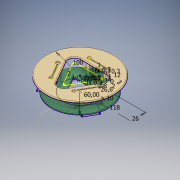
# Autodesk Inventor part: Stewart-Plate-inside
Saved by Autodesk Inventor 2018.2 (Build 222227000, 227)
## iProperties
Created: 2018-02-18
Part Number: Stewart-Plate-inside
Material: Generisch
Document SubType Name: Modeling
Designer: JochenAlt
Density: 1 g/cm^3
Appearance: Vorgabe
Author: JochenAlt
Autodesk Inventor part; units mm, degrees
ref_plane "YZ Plane" through (0, 0, 0) normal (1, 0, 0) x (0, 1, 0)
ref_plane "XZ Plane" through (0, 0, 0) normal (0, 1, 0) x (-1, 0, 0)
sketch "Skizze1" plane through (0, 0, 0) normal (0, 0, 1) x (1, 0, 0)
  line L0 (-9.8, 0) -> (9.8, 0) construction
  line L1 (-7, 36) -> (7, 36)
  line L2 (7, 36) -> (7, 33)
  line L3 (7, 33) -> (-7, 33)
  line L4 (-7, 33) -> (-7, 36)
  line L5 (1.5, 33) -> (-1.5, 33)
  line L6 (-1.5, 33) -> (-1.5, 28)
  line L7 (-1.5, 28) -> (1.5, 28)
  line L8 (1.5, 28) -> (1.5, 33)
  line L9 (0, 43.2) -> (0, -7.2) construction
  point P0 (0, 0)
  dimension "d10" = 3
  dimension "d14" = 14
  dimension "d23" = 5
  constraints: 16 end point, 4 parallel, 3 perpendicular, 2 horizontal, 2 point on line, 1 midpoint, 1 other
  measures "d10" distance between parallel lines of L3 L1
  measures "d14" distance between parallel lines of L2 L4
  measures "d23" distance between parallel lines of L3 L7
extrude "Extrusion3" add sketch "Skizze1" against normal blind 7
fillet "Rundung1" radius 4 2 edges at (-7, 34.5, -7) (7, 34.5, -7)
sketch "Skizze2" plane through (-7, 36, 0) normal (0, 1, 0) x (1, 0, 0)
  circle A0 centre (3, 4) radius 1.1
  circle A1 centre (11, 4) radius 1.1
  line L0 (7, 0) -> (7, 7) construction
  line L1 (43, 0) -> (-27, 0) construction
  line L2 (-1.6221, 4) -> (19.0112, 4) construction
  line L3 (0, 7) -> (14, 7) construction
  line L4 (0, 0) -> (0, 7) projected
  point P0 (4, 7)
  point P1 (10, 7)
  point P2 (0, 3)
  dimension "d16" = 2.2
  dimension "d20" = 3
  dimension "d21" = 3
  constraints: 4 end point, 2 centre point, 1 equal radius, 1 horizontal, 1 midpoint, 1 point on line, 1 symmetric about line, 1 vertical
  measures "d16" diameter of A0
  measures "d20" distance between parallel lines of L3 L2
  measures "d21" distance from line of L4 A0.centre
extrude "Extrusion4" cut sketch "Skizze2" against normal up to next
chamfer "Fase1" distance 5 distance2 7 1 edges at (0, 28, -7) measured on face at (0, 28.5, -7)
pattern_circular "Runde Anordnung1" count 3 over 360 about axis through (0, 0, -10) along (0, 0, 1) of "Extrusion3", "Extrusion4", "Fase1", "Rundung1"
sketch "Skizze3" plane through (0, 0, 0) normal (0, 0, 1) x (1, 0, 0)
  line L0 (0, 73.7285) -> (0, -70.6214) construction
  circle A0 centre (0, 0) radius 50
  line L1 (23.7291, 15.7) -> (-23.7291, 15.7)
  line L2 (-25.4611, 12.7) -> (-1.7321, -28.4)
  line L3 (25.4611, 12.7) -> (1.7321, -28.4)
  line L4 (-11.5394, 6.6623) -> (13.5966, -7.85) construction
  line L5 (27.1932, 15.7) -> (-13.5966, -7.85) construction
  line L6 (0.15, 52.6) -> (12.15, 52.6) construction
  line L7 (12.15, 52.6) -> (12.15, 26) construction
  line L8 (12.15, 26) -> (0.15, 26) construction
  line L9 (0.15, 26) -> (0.15, 52.6) construction
  line L10 (-0.15, 52.6) -> (-12.15, 52.6) construction
  line L11 (-12.15, 52.6) -> (-12.15, 26) construction
  line L12 (-12.15, 26) -> (-0.15, 26) construction
  line L13 (-0.15, 26) -> (-0.15, 52.6) construction
  line L14 (11.45, 25.7) -> (-11.45, 25.7)
  arc A1 (-23.7291, 15.7) -> (-25.4611, 12.7) centre (-23.7291, 13.7) ccw
  arc A2 (-1.7321, -28.4) -> (1.7321, -28.4) centre (0, -27.4) ccw
  arc A3 (25.4611, 12.7) -> (23.7291, 15.7) centre (23.7291, 13.7) ccw
  line L15 (-12.45, 31.5) -> (12.45, 31.5) construction
  line L16 (12.45, 32.7) -> (-12.45, 32.7) construction
  line L17 (-12.45, 31.2) -> (12.45, 31.2)
  line L18 (-12.45, 33) -> (12.45, 33)
  line L19 (-12.45, 26.7) -> (-12.45, 51.9)
  line L20 (-11.45, 52.9) -> (11.45, 52.9)
  line L21 (12.45, 51.9) -> (12.45, 26.7)
  arc A4 (-11.45, 52.9) -> (-12.45, 51.9) centre (-11.45, 51.9) ccw
  arc A5 (12.45, 51.9) -> (11.45, 52.9) centre (11.45, 51.9) ccw
  arc A6 (11.45, 25.7) -> (12.45, 26.7) centre (11.45, 26.7) ccw
  arc A7 (-12.45, 26.7) -> (-11.45, 25.7) centre (-11.45, 26.7) ccw
  line L22 (-12.45, 35.15) -> (12.45, 35.15) construction
  circle A8 centre (0, 0) radius 36.7791 construction
  circle A9 centre (-16.6, 32.8198) radius 2.15 construction
  line L23 (-14.3846, 33.9403) -> (-14.5219, 31.4615)
  line L24 (-14.5219, 31.4615) -> (-16.7373, 30.341)
  line L25 (-16.7373, 30.341) -> (-18.8154, 31.6993)
  line L26 (-18.8154, 31.6993) -> (-18.6781, 34.1781)
  line L27 (-18.6781, 34.1781) -> (-16.4627, 35.2986)
  line L28 (-16.4627, 35.2986) -> (-14.3846, 33.9403)
  line L29 (-16.6, 32.8198) -> (-17.5704, 34.7383) construction
  line L30 (-16.6, 32.8198) -> (0, 0) construction
  line L31 (0, 0) -> (16.6, 32.8198) construction
  circle A10 centre (16.6, 32.8198) radius 2.15 construction
  line L32 (18.8154, 31.6993) -> (16.7373, 30.341)
  line L33 (16.7373, 30.341) -> (14.5219, 31.4615)
  line L34 (14.5219, 31.4615) -> (14.3846, 33.9403)
  line L35 (14.3846, 33.9403) -> (16.4627, 35.2986)
  line L36 (16.4627, 35.2986) -> (18.6781, 34.1781)
  line L37 (18.6781, 34.1781) -> (18.8154, 31.6993)
  line L38 (16.6, 32.8198) -> (17.5704, 34.7383) construction
  arc A11 (16.6, 28.6698) -> (16.6, 36.9698) centre (16.6, 32.8198) ccw
  line L39 (-12.45, 36.9698) -> (-12.45, 28.6698)
  line L40 (-12.45, 28.6698) -> (-16.6, 28.6698)
  arc A12 (-16.6, 36.9698) -> (-16.6, 28.6698) centre (-16.6, 32.8198) ccw
  line L41 (12.45, 36.9698) -> (12.45, 28.6698)
  line L42 (16.6, 36.9698) -> (12.45, 36.9698)
  line L43 (16.6, 28.6698) -> (12.45, 28.6698)
  line L44 (-12.45, 36.9698) -> (-16.6, 36.9698)
  circle A13 centre (16.6, 32.8198) radius 4.15 construction
  circle A14 centre (-16.6, 32.8198) radius 4.15 construction
  circle A15 centre (16.6, 32.8198) radius 1.4
  circle A16 centre (-16.6, 32.8198) radius 1.4
  line L45 (-16.8979, -24.132) -> (-38.7217, -36.732)
  line L46 (-40.0877, -36.366) -> (-51.5377, -16.534)
  arc A17 (-40.0877, -36.366) -> (-38.7217, -36.732) centre (-39.2217, -35.866) ccw
  arc A18 (-16.8979, -24.132) -> (-16.5319, -22.766) centre (-17.3979, -23.266) ccw
  line L47 (-27.9819, -2.934) -> (-16.5319, -22.766)
  line L48 (-20.795, -26.382) -> (-33.245, -4.818)
  line L49 (-22.3538, -27.282) -> (-34.8038, -5.718)
  line L50 (-51.1717, -15.168) -> (-29.3479, -2.568)
  line L51 (-40.3168, -4.1089) -> (-38.2418, -7.7029)
  line L52 (-36.5855, -4.5127) -> (-38.8008, -3.3922)
  line L53 (-34.5074, -3.1544) -> (-36.5855, -4.5127)
  circle A19 centre (-36.7228, -2.0339) radius 2.15 construction
  line L54 (-33.1288, 0.0411) -> (-31.0538, -3.5529)
  arc A20 (-33.1288, 0.0411) -> (-40.3168, -4.1089) centre (-36.7228, -2.0339) ccw
  line L55 (-36.8601, 0.4449) -> (-34.6447, -0.6756)
  circle A21 centre (-36.7228, -2.0339) radius 1.4
  line L56 (0, 0) -> (-36.7228, -2.0339) construction
  line L57 (-34.6447, -0.6756) -> (-34.5074, -3.1544)
  line L58 (-38.8008, -3.3922) -> (-38.9381, -0.9134)
  line L59 (-38.9381, -0.9134) -> (-36.8601, 0.4449)
  line L60 (-22.2008, -29.4276) -> (-19.9855, -28.3071)
  line L61 (-18.6038, -25.1169) -> (-16.5288, -28.7109)
  line L62 (-25.7918, -29.2669) -> (-18.6038, -25.1169)
  line L63 (-22.3381, -31.9064) -> (-22.2008, -29.4276)
  circle A22 centre (-20.1228, -30.7859) radius 1.4
  line L64 (-25.7918, -29.2669) -> (-23.7168, -32.8609)
  circle A23 centre (-20.1228, -30.7859) radius 4.15 construction
  line L65 (-17.9074, -29.6654) -> (-18.0447, -32.1442)
  line L66 (-19.9855, -28.3071) -> (-17.9074, -29.6654)
  line L67 (-18.0447, -32.1442) -> (-20.2601, -33.2647)
  arc A24 (-23.7168, -32.8609) -> (-16.5288, -28.7109) centre (-20.1228, -30.7859) ccw
  line L68 (-20.2601, -33.2647) -> (-22.3381, -31.9064)
  line L69 (-38.2418, -7.7029) -> (-31.0538, -3.5529)
  arc A25 (-27.9819, -2.934) -> (-29.3479, -2.568) centre (-28.8479, -3.434) ccw
  arc A26 (-51.1717, -15.168) -> (-51.5377, -16.534) centre (-50.6717, -16.034) ccw
  line L70 (29.3479, -2.568) -> (51.1717, -15.168)
  line L71 (51.5377, -16.534) -> (40.0877, -36.366)
  arc A27 (51.5377, -16.534) -> (51.1717, -15.168) centre (50.6717, -16.034) ccw
  arc A28 (29.3479, -2.568) -> (27.9819, -2.934) centre (28.8479, -3.434) ccw
  line L72 (16.5319, -22.766) -> (27.9819, -2.934)
  line L73 (33.245, -4.818) -> (20.795, -26.382)
  line L74 (34.8038, -5.718) -> (22.3538, -27.282)
  line L75 (38.7217, -36.732) -> (16.8979, -24.132)
  line L76 (23.7168, -32.8609) -> (25.7918, -29.2669)
  line L77 (22.2008, -29.4276) -> (22.3381, -31.9064)
  line L78 (19.9855, -28.3071) -> (22.2008, -29.4276)
  circle A29 centre (20.1228, -30.7859) radius 2.15 construction
  line L79 (16.5288, -28.7109) -> (18.6038, -25.1169)
  arc A30 (16.5288, -28.7109) -> (23.7168, -32.8609) centre (20.1228, -30.7859) ccw
  line L80 (18.0447, -32.1442) -> (17.9074, -29.6654)
  circle A31 centre (20.1228, -30.7859) radius 1.4
  line L81 (0, 0) -> (20.1228, -30.7859) construction
  line L82 (17.9074, -29.6654) -> (19.9855, -28.3071)
  line L83 (22.3381, -31.9064) -> (20.2601, -33.2647)
  line L84 (20.2601, -33.2647) -> (18.0447, -32.1442)
  line L85 (36.5855, -4.5127) -> (34.5074, -3.1544)
  line L86 (31.0538, -3.5529) -> (33.1288, 0.0411)
  line L87 (38.2418, -7.7029) -> (31.0538, -3.5529)
  line L88 (38.8008, -3.3922) -> (36.5855, -4.5127)
  circle A32 centre (36.7228, -2.0339) radius 1.4
  line L89 (38.2418, -7.7029) -> (40.3168, -4.1089)
  circle A33 centre (36.7228, -2.0339) radius 4.15 construction
  line L90 (34.6447, -0.6756) -> (36.8601, 0.4449)
  line L91 (34.5074, -3.1544) -> (34.6447, -0.6756)
  line L92 (36.8601, 0.4449) -> (38.9381, -0.9134)
  arc A34 (40.3168, -4.1089) -> (33.1288, 0.0411) centre (36.7228, -2.0339) ccw
  line L93 (38.9381, -0.9134) -> (38.8008, -3.3922)
  line L94 (25.7918, -29.2669) -> (18.6038, -25.1169)
  arc A35 (16.5319, -22.766) -> (16.8979, -24.132) centre (17.3979, -23.266) ccw
  arc A36 (38.7217, -36.732) -> (40.0877, -36.366) centre (39.2217, -35.866) ccw
  point P0 (-27.1932, 15.7)
  point P1 (0, -31.4)
  point P2 (19.75, 15.7)
  point P3 (-14.2556, 15.7)
  point P4 (-15.9349, -3.8)
  point P5 (11.2583, -11.9)
  point P6 (-4.5899, -23.45)
  point P7 (-15.4237, 34.6195)
  point P8 (18.7467, 32.9387)
  point P9 (-24.2158, -28.357)
  point P10 (-22.094, -27.132)
  point P11 (-21.0548, -26.532)
  point P12 (-36.6658, -6.793)
  point P13 (-34.544, -5.568)
  point P14 (-33.5048, -4.968)
  point P15 (-37.8991, -0.2342)
  point P16 (-38.8695, -2.1528)
  point P17 (-22.2695, -30.667)
  point P18 (-21.2991, -32.5856)
  point P19 (36.6658, -6.793)
  point P20 (34.544, -5.568)
  point P21 (33.5048, -4.968)
  point P22 (24.2158, -28.357)
  point P23 (22.094, -27.132)
  point P24 (21.0548, -26.532)
  point P25 (19.1524, -32.7045)
  point P26 (21.2991, -32.5856)
  point P27 (37.6932, -3.9524)
  point P28 (38.8695, -2.1528)
  dimension "d140" = 60
  dimension "d146" = 0.3
  dimension "d147" = 26.6
  dimension "d148" = 12
  dimension "d150" = 0.3
  dimension "d160" = 10
  dimension "d164" = 26
  dimension "d184" = 2
  dimension "d189" = 100
  dimension "d199" = 5.5
  dimension "d200" = 1.2
  dimension "d201" = 0.3
  dimension "d202" = 0.3
  dimension "d203" = 0.3
  dimension "d204" = 0.3
  dimension "d205" = 1
  dimension "d211" = 4.3
  dimension "d213" = 0
  dimension "d214" = 2
  dimension "d227" = 2.8
  dimension "d230" = 360
  constraints: 188 end point, 54 point on circle, 48 point on line, 37 centre point, 21 tangent, 11 coincident, 10 midpoint, 8 equal radius, 6 parallel, 5 horizontal, 4 collinear, 4 perpendicular, 2 symmetric about line, 2 vertical, 298 other
  measures "d140" angle of L3 L1
  measures "d146" distance between parallel lines of L9 L13
  measures "d147" distance between parallel lines of L8 L6
  measures "d148" distance between parallel lines of L7 L9
  measures "d150" distance between parallel lines of L14 L8
  measures "d160" distance between parallel lines of L1 L14
  measures "d164" distance from line of point (0, 0) L8
  measures "d184" radius of A1
  measures "d189" diameter of A0
  measures "d199" distance between parallel lines of L15 L12
  measures "d200" distance between parallel lines of L16 L15
  measures "d201" distance between parallel lines of L17 L15
  measures "d202" distance between parallel lines of L16 L18
  measures "d203" distance between parallel lines of L6 L20
  measures "d204" distance between parallel lines of L11 L19
  measures "d205" radius of A4
  measures "d211" diameter of A9
  measures "d213" distance between parallel lines of L21 L41
  measures "d214" radial gap between concentric circles of A13 A10
  measures "d227" diameter of A15
extrude "Extrusion11" add sketch "Skizze3" along normal blind 2.5 contours A0 L70 L89 A34 L86 A28 L72 A35 L75 L79 A30 L76 L45 L64 A24 L61 A18 L47 A25 L50 L54 A20 L51 L19 L44 A12 L40 A7 L14 A6 L21 L43 A11 L42 | L21 L18 L19 A0 | A0 L75 L74 L70 | L42 A11 L43 L21 | L70 L86 A34 L89 | L50 L49 L45 A0 | L19 L40 A12 L44 | L76 A30 L79 L75 | L51 A20 L54 L50 | L21 A6 L14 A7 L19 L17 | L45 L61 A24 L64 | L73 L75 A35 L72 A28 L70 | L50 A25 L47 A18 L45 L48 | L23 L24 L25 L26 L27 L28 | L32 L33 L34 L35 L36 L37 | L52 L58 L59 L55 L57 L53 | L60 L66 L65 L67 L68 L63 | L77 L83 L84 L80 L82 L78 | L85 L91 L90 L92 L93 L88
extrude "Extrusion9" cut sketch "Skizze3" against normal blind 1 from surface at 2.5 contours L21 L18 L19 A0 | A0 L19 A4 L20 A5 L21 | L70 A27 L71 A36 L75 A0 | A0 L75 L74 L70 | L50 L49 L45 A0 | A0 L45 A17 L46 A26 L50 | L21 A6 L14 A7 L19 L17 | L73 L75 A35 L72 A28 L70 | L50 A25 L47 A18 L45 L48 | A3 L3 A2 L2 A1 L1
fillet "Rundung4" radius 1 17 edges at (0, -50, 2.5) (49.5385, -6.7778, 2.5) (39.5127, 30.639, 2.5) (-43.3013, 25, 2.5) (-50, 0, 0) (25.4611, 14.7, 2.5) (13.5966, -7.85, 2.5) (0, -29.4, 2.5) (-13.5966, -7.85, 2.5) (-25.4611, 14.7, 2.5) (0, 15.7, 2.5) (-25.4611, 14.7, 0) (-13.5966, -7.85, 0) (0, -29.4, 0) (13.5966, -7.85, 0) (25.4611, 14.7, 0) (0, 15.7, 0)
fillet "Rundung4" radius 0.75 7 edges at (-12.45, 40.7126, 1.5) (-12.1571, 25.9929, 1.5) (0, 25.7, 1.5) (12.1571, 25.9929, 1.5) (12.45, 28.95, 1.5) (-12.45, 28.95, 1.5) (12.45, 40.7126, 1.5)
extrude "Extrusion14" add sketch "Skizze3" along normal blind 13 contours L42 A11 L43 L21 | L70 L86 A34 L89 | L19 L40 A12 L44 | L76 A30 L79 L75 | L51 A20 L54 L50 | L45 L61 A24 L64 | L23 L24 L25 L26 L27 L28 | L32 L33 L34 L35 L36 L37 | L52 L58 L59 L55 L57 L53 | L60 L66 L65 L67 L68 L63 | L77 L83 L84 L80 L82 L78 | L85 L91 L90 L92 L93 L88
extrude "Extrusion15" cut sketch "Skizze3" against normal blind 6 from surface at 13 contours L23 L24 L25 L26 L27 L28 | L32 L33 L34 L35 L36 L37 | A15 | A16 | L52 L58 L59 L55 L57 L53 | L60 L66 L65 L67 L68 L63 | L77 L83 L84 L80 L82 L78 | L85 L91 L90 L92 L93 L88
ref_plane "Arbeitsebene1" through (0, 0, 24.5) normal (0, 0, 1) x (1, 0, 0)
sketch "Skizze8" plane through (0, 0, 24.5) normal (0, 0, 1) x (1, 0, 0)
  circle A0 centre (36.7228, -2.0339) radius 1.4 projected
  circle A1 centre (20.1228, -30.7859) radius 1.4 projected
  circle A2 centre (-20.1228, -30.7859) radius 1.4 projected
  circle A3 centre (-36.7228, -2.0339) radius 1.4 projected
  circle A4 centre (-16.6, 32.8198) radius 1.4 projected
  circle A5 centre (16.6, 32.8198) radius 1.4 projected
  line L0 (18.6781, 34.1781) -> (18.8154, 31.6993) projected
  line L1 (16.4627, 35.2986) -> (18.6781, 34.1781) projected
  line L2 (14.3846, 33.9403) -> (16.4627, 35.2986) projected
  line L3 (14.5219, 31.4615) -> (14.3846, 33.9403) projected
  line L4 (16.7373, 30.341) -> (14.5219, 31.4615) projected
  line L5 (18.8154, 31.6993) -> (16.7373, 30.341) projected
  circle A6 centre (-16.6, 32.8198) radius 1.4 projected
  line L6 (-16.4627, 35.2986) -> (-14.3846, 33.9403) projected
  line L7 (-18.6781, 34.1781) -> (-16.4627, 35.2986) projected
  line L8 (-18.8154, 31.6993) -> (-18.6781, 34.1781) projected
  line L9 (-16.7373, 30.341) -> (-18.8154, 31.6993) projected
  line L10 (-14.5219, 31.4615) -> (-16.7373, 30.341) projected
  line L11 (-14.3846, 33.9403) -> (-14.5219, 31.4615) projected
  circle A7 centre (-36.7228, -2.0339) radius 1.4 projected
  line L12 (-34.6447, -0.6756) -> (-34.5074, -3.1544) projected
  line L13 (-36.8601, 0.4449) -> (-34.6447, -0.6756) projected
  line L14 (-38.9381, -0.9134) -> (-36.8601, 0.4449) projected
  line L15 (-38.8008, -3.3922) -> (-38.9381, -0.9134) projected
  line L16 (-36.5855, -4.5127) -> (-38.8008, -3.3922) projected
  line L17 (-34.5074, -3.1544) -> (-36.5855, -4.5127) projected
  circle A8 centre (36.7228, -2.0339) radius 1.4 projected
  line L18 (38.8008, -3.3922) -> (36.5855, -4.5127) projected
  line L19 (38.9381, -0.9134) -> (38.8008, -3.3922) projected
  line L20 (36.8601, 0.4449) -> (38.9381, -0.9134) projected
  line L21 (34.6447, -0.6756) -> (36.8601, 0.4449) projected
  line L22 (34.5074, -3.1544) -> (34.6447, -0.6756) projected
  line L23 (36.5855, -4.5127) -> (34.5074, -3.1544) projected
  circle A9 centre (20.1228, -30.7859) radius 1.4 projected
  line L24 (17.9074, -29.6654) -> (19.9855, -28.3071) projected
  line L25 (18.0447, -32.1442) -> (17.9074, -29.6654) projected
  line L26 (20.2601, -33.2647) -> (18.0447, -32.1442) projected
  line L27 (22.3381, -31.9064) -> (20.2601, -33.2647) projected
  line L28 (22.2008, -29.4276) -> (22.3381, -31.9064) projected
  line L29 (19.9855, -28.3071) -> (22.2008, -29.4276) projected
  circle A10 centre (-20.1228, -30.7859) radius 1.4 projected
  line L30 (-22.3381, -31.9064) -> (-22.2008, -29.4276) projected
  line L31 (-20.2601, -33.2647) -> (-22.3381, -31.9064) projected
  line L32 (-18.0447, -32.1442) -> (-20.2601, -33.2647) projected
  line L33 (-17.9074, -29.6654) -> (-18.0447, -32.1442) projected
  line L34 (-19.9855, -28.3071) -> (-17.9074, -29.6654) projected
  line L35 (-22.2008, -29.4276) -> (-19.9855, -28.3071) projected
  line L36 (-22.3381, -31.9064) -> (-22.2008, -29.4276) projected
  line L37 (-22.2008, -29.4276) -> (-19.9855, -28.3071) projected
  line L38 (-19.9855, -28.3071) -> (-17.9074, -29.6654) projected
  line L39 (-17.9074, -29.6654) -> (-18.0447, -32.1442) projected
  line L40 (-18.0447, -32.1442) -> (-20.2601, -33.2647) projected
  line L41 (-20.2601, -33.2647) -> (-22.3381, -31.9064) projected
  line L42 (-18.6038, -25.1169) -> (-25.7918, -29.2669) projected
  line L43 (-25.7918, -29.2669) -> (-23.7168, -32.8609) projected
  arc A11 (-23.7168, -32.8609) -> (-16.5288, -28.7109) centre (-20.1228, -30.7859) ccw projected
  line L44 (-16.5288, -28.7109) -> (-18.6038, -25.1169) projected
  line L45 (-34.6447, -0.6756) -> (-34.5074, -3.1544) projected
  line L46 (-34.5074, -3.1544) -> (-36.5855, -4.5127) projected
  line L47 (-36.5855, -4.5127) -> (-38.8008, -3.3922) projected
  line L48 (-38.8008, -3.3922) -> (-38.9381, -0.9134) projected
  line L49 (-38.9381, -0.9134) -> (-36.8601, 0.4449) projected
  line L50 (-36.8601, 0.4449) -> (-34.6447, -0.6756) projected
  line L51 (-40.3168, -4.1089) -> (-38.2418, -7.7029) projected
  line L52 (-38.2418, -7.7029) -> (-31.0538, -3.5529) projected
  line L53 (-31.0538, -3.5529) -> (-33.1288, 0.0411) projected
  arc A12 (-33.1288, 0.0411) -> (-40.3168, -4.1089) centre (-36.7228, -2.0339) ccw projected
  line L54 (17.9074, -29.6654) -> (19.9855, -28.3071) projected
  line L55 (19.9855, -28.3071) -> (22.2008, -29.4276) projected
  line L56 (22.2008, -29.4276) -> (22.3381, -31.9064) projected
  line L57 (22.3381, -31.9064) -> (20.2601, -33.2647) projected
  line L58 (20.2601, -33.2647) -> (18.0447, -32.1442) projected
  line L59 (18.0447, -32.1442) -> (17.9074, -29.6654) projected
  line L60 (23.7168, -32.8609) -> (25.7918, -29.2669) projected
  line L61 (25.7918, -29.2669) -> (18.6038, -25.1169) projected
  line L62 (18.6038, -25.1169) -> (16.5288, -28.7109) projected
  arc A13 (16.5288, -28.7109) -> (23.7168, -32.8609) centre (20.1228, -30.7859) ccw projected
  line L63 (38.8008, -3.3922) -> (36.5855, -4.5127) projected
  line L64 (36.5855, -4.5127) -> (34.5074, -3.1544) projected
  line L65 (34.5074, -3.1544) -> (34.6447, -0.6756) projected
  line L66 (34.6447, -0.6756) -> (36.8601, 0.4449) projected
  line L67 (36.8601, 0.4449) -> (38.9381, -0.9134) projected
  line L68 (38.9381, -0.9134) -> (38.8008, -3.3922) projected
  line L69 (31.0538, -3.5529) -> (38.2418, -7.7029) projected
  line L70 (38.2418, -7.7029) -> (40.3168, -4.1089) projected
  arc A14 (40.3168, -4.1089) -> (33.1288, 0.0411) centre (36.7228, -2.0339) ccw projected
  line L71 (33.1288, 0.0411) -> (31.0538, -3.5529) projected
  line L72 (18.6781, 34.1781) -> (18.8154, 31.6993) projected
  line L73 (18.8154, 31.6993) -> (16.7373, 30.341) projected
  line L74 (16.7373, 30.341) -> (14.5219, 31.4615) projected
  line L75 (14.5219, 31.4615) -> (14.3846, 33.9403) projected
  line L76 (14.3846, 33.9403) -> (16.4627, 35.2986) projected
  line L77 (16.4627, 35.2986) -> (18.6781, 34.1781) projected
  line L78 (12.45, 36.9698) -> (12.45, 28.6698) projected
  line L79 (12.45, 28.6698) -> (16.6, 28.6698) projected
  arc A15 (16.6, 28.6698) -> (16.6, 36.9698) centre (16.6, 32.8198) ccw projected
  line L80 (16.6, 36.9698) -> (12.45, 36.9698) projected
  line L81 (-16.4627, 35.2986) -> (-14.3846, 33.9403) projected
  line L82 (-14.3846, 33.9403) -> (-14.5219, 31.4615) projected
  line L83 (-14.5219, 31.4615) -> (-16.7373, 30.341) projected
  line L84 (-16.7373, 30.341) -> (-18.8154, 31.6993) projected
  line L85 (-18.8154, 31.6993) -> (-18.6781, 34.1781) projected
  line L86 (-18.6781, 34.1781) -> (-16.4627, 35.2986) projected
  line L87 (-12.45, 28.6698) -> (-12.45, 36.9698) projected
  line L88 (-12.45, 36.9698) -> (-16.6, 36.9698) projected
  arc A16 (-16.6, 36.9698) -> (-16.6, 28.6698) centre (-16.6, 32.8198) ccw projected
  line L89 (-16.6, 28.6698) -> (-12.45, 28.6698) projected
  circle A17 centre (0, 0) radius 59
  line L90 (51.5377, -16.534) -> (40.0877, -36.366) projected
  arc A18 (38.7217, -36.732) -> (40.0877, -36.366) centre (39.2217, -35.866) ccw projected
  line L91 (38.7217, -36.732) -> (16.8979, -24.132) projected
  line L92 (34.8038, -5.718) -> (22.3538, -27.282) projected
  line L93 (33.245, -4.818) -> (20.795, -26.382) projected
  line L94 (16.5319, -22.766) -> (27.9819, -2.934) projected
  arc A19 (16.5319, -22.766) -> (16.8979, -24.132) centre (17.3979, -23.266) ccw projected
  line L95 (29.3479, -2.568) -> (51.1717, -15.168) projected
  arc A20 (29.3479, -2.568) -> (27.9819, -2.934) centre (28.8479, -3.434) ccw projected
  arc A21 (51.5377, -16.534) -> (51.1717, -15.168) centre (50.6717, -16.034) ccw projected
  line L96 (-27.9819, -2.934) -> (-16.5319, -22.766) projected
  arc A22 (-16.8979, -24.132) -> (-16.5319, -22.766) centre (-17.3979, -23.266) ccw projected
  line L97 (-16.8979, -24.132) -> (-38.7217, -36.732) projected
  arc A23 (-40.0877, -36.366) -> (-38.7217, -36.732) centre (-39.2217, -35.866) ccw projected
  line L98 (-40.0877, -36.366) -> (-51.5377, -16.534) projected
  arc A24 (-51.1717, -15.168) -> (-51.5377, -16.534) centre (-50.6717, -16.034) ccw projected
  line L99 (-51.1717, -15.168) -> (-29.3479, -2.568) projected
  arc A25 (-27.9819, -2.934) -> (-29.3479, -2.568) centre (-28.8479, -3.434) ccw projected
  line L100 (-12.45, 26.7) -> (-12.45, 51.9) projected
  line L101 (-11.45, 52.9) -> (11.45, 52.9) projected
  line L102 (12.45, 51.9) -> (12.45, 26.7) projected
  arc A26 (12.45, 51.9) -> (11.45, 52.9) centre (11.45, 51.9) ccw projected
  arc A27 (-11.45, 52.9) -> (-12.45, 51.9) centre (-11.45, 51.9) ccw projected
  arc A28 (11.45, 25.7) -> (12.45, 26.7) centre (11.45, 26.7) ccw projected
  line L103 (11.45, 25.7) -> (-11.45, 25.7) projected
  arc A29 (-12.45, 26.7) -> (-11.45, 25.7) centre (-11.45, 26.7) ccw projected
  line L104 (-12.45, 33) -> (12.45, 33) projected
  line L105 (-12.45, 31.2) -> (12.45, 31.2) projected
  line L106 (-20.795, -26.382) -> (-33.245, -4.818) projected
  line L107 (-22.3538, -27.282) -> (-34.8038, -5.718) projected
  line L108 (25.4611, 12.7) -> (1.7321, -28.4) projected
  arc A30 (-1.7321, -28.4) -> (1.7321, -28.4) centre (0, -27.4) ccw projected
  line L109 (-25.4611, 12.7) -> (-1.7321, -28.4) projected
  arc A31 (25.4611, 12.7) -> (23.7291, 15.7) centre (23.7291, 13.7) ccw projected
  line L110 (23.7291, 15.7) -> (-23.7291, 15.7) projected
  arc A32 (-23.7291, 15.7) -> (-25.4611, 12.7) centre (-23.7291, 13.7) ccw projected
  line L111 (-23.7291, 24.7) -> (23.7291, 24.7)
  arc A33 (33.2554, 8.2) -> (23.7291, 24.7) centre (23.7291, 13.7) ccw
  line L112 (33.2554, 8.2) -> (9.5263, -32.9)
  arc A34 (-9.5263, -32.9) -> (9.5263, -32.9) centre (0, -27.4) ccw
  line L113 (-9.5263, -32.9) -> (-33.2554, 8.2)
  arc A35 (-23.7291, 24.7) -> (-33.2554, 8.2) centre (-23.7291, 13.7) ccw
  dimension "d236" = 118
  dimension "d251" = 1
  constraints: 6 end point, 6 point on circle, 4 centre point, 1 coincident, 5 other
  measures "d236" diameter of A17
  measures "d251" distance between parallel lines of L103 L111
extrude "Extrusion17" add sketch "Skizze8" along normal blind 2 separate body contours L0 L5 L4 L3 L2 L1 | L6 L11 L10 L9 L8 L7 | L12 L17 L16 L15 L14 L13 | L18 L23 L22 L21 L20 L19 | L24 L29 L28 L27 L26 L25 | L30 L35 L34 L33 L32 L31 | L44 A11 L43 L42 | L42 L106 L52 L99 A25 L96 A22 L97 | L42 L97 A23 L98 A24 L99 L52 L107 | L52 L51 A12 L53 | A13 L62 L61 L60 | L61 L92 L69 L95 A21 L90 A18 L91 | L91 A19 L94 A20 L95 L69 L93 L61 | L69 L71 A14 L70 | L80 A15 L79 L78 | L78 L104 L87 L100 A27 L101 A26 L102 | L78 L102 A28 L103 A29 L100 L87 L105 | L87 L89 A16 L88 | A17
extrude "Extrusion20" cut sketch "Skizze8" along normal blind 1 contours A0 | L42 L106 L52 L99 A25 L96 A22 L97 | L42 L107 L52 L106 | L42 L97 A23 L98 A24 L99 L52 L107 | L61 L92 L69 L95 A21 L90 A18 L91 | L61 L93 L69 L92 | L91 A19 L94 A20 L95 L69 L93 L61 | L78 L104 L87 L100 A27 L101 A26 L102 | L78 L105 L87 L104 | L78 L102 A28 L103 A29 L100 L87 L105 bodies 1 2
extrude "Extrusion18" add sketch "Skizze8" against normal up to surface (11.5 mm away) contours L6 L11 L10 L9 L8 L7 | L12 L17 L16 L15 L14 L13 | L24 L29 L28 L27 L26 L25 | L30 L35 L34 L33 L32 L31 | L44 A11 L43 L42 | L52 L51 A12 L53 | A13 L62 L61 L60 | L69 L71 A14 L70 | L80 A15 L79 L78 | L87 L89 A16 L88 bodies 2
extrude "Extrusion19" cut sketch "Skizze8" along normal blind 6 from surface at -11.5 contours L0 L5 L4 L3 L2 L1 | L6 L11 L10 L9 L8 L7 | L12 L17 L16 L15 L14 L13 | L18 L23 L22 L21 L20 L19 | L24 L29 L28 L27 L26 L25 | L30 L35 L34 L33 L32 L31 bodies 1
fillet "Rundung6" radius 1 14 edges at (-59, 0, 24.5) (-59, 0, 26.5) (33.2554, 19.2, 26.5) (21.3908, -12.35, 26.5) (0, -38.4, 26.5) (-21.3908, -12.35, 26.5) (-33.2554, 19.2, 26.5) (0, 24.7, 26.5) (-33.2554, 19.2, 24.5) (-21.3908, -12.35, 24.5) (0, -38.4, 24.5) (21.3908, -12.35, 24.5) (33.2554, 19.2, 24.5) (0, 24.7, 24.5)
fillet "Rundung6" radius 0.75 30 edges at (51.6376, -15.7752, 25.5) (45.8127, -26.45, 25.5) (39.4805, -36.8319, 25.5) (30.5378, -32.007, 25.5) (42.9878, -10.443, 25.5) (28.5891, -2.4681, 25.5) (22.2569, -12.85, 25.5) (16.432, -23.5248, 25.5) (18.8464, -25.257, 25.5) (31.2964, -3.693, 25.5) (-51.6376, -15.7752, 25.5) (-45.8127, -26.45, 25.5) (-39.4805, -36.8319, 25.5) (-30.5378, -32.007, 25.5) (-42.9878, -10.443, 25.5) (-31.2964, -3.693, 25.5) (-22.2569, -12.85, 25.5) (-16.432, -23.5248, 25.5) (-18.8464, -25.257, 25.5) (-28.5891, -2.4681, 25.5) (12.1571, 25.9929, 25.5) (0, 25.7, 25.5) (-12.1571, 25.9929, 25.5) (-12.45, 28.95, 25.5) (12.45, 28.95, 25.5) (12.1571, 52.6071, 25.5) (0, 52.9, 25.5) (-12.1571, 52.6071, 25.5) (-12.45, 42.45, 25.5) (12.45, 42.45, 25.5)
sketch "Skizze9" plane through (0, 0, 26.5) normal (0, 0, 1) x (1, 0, 0)
  circle A0 centre (-20.1228, -30.7859) radius 2.75
  circle A1 centre (20.1228, -30.7859) radius 2.75
  circle A2 centre (36.7228, -2.0339) radius 2.75
  circle A3 centre (16.6, 32.8198) radius 2.75
  circle A4 centre (-16.6, 32.8198) radius 2.75
  circle A5 centre (-36.7228, -2.0339) radius 3.2422
  point P0 (0, 0)
  dimension "d248" = 5.5
  constraints: 6 centre point, 6 coincident, 4 equal radius
  measures "d248" diameter of A0
extrude "Extrusion21" cut sketch "Skizze9" against normal blind 2 bodies 2
equation "\"d21\" = d20"
